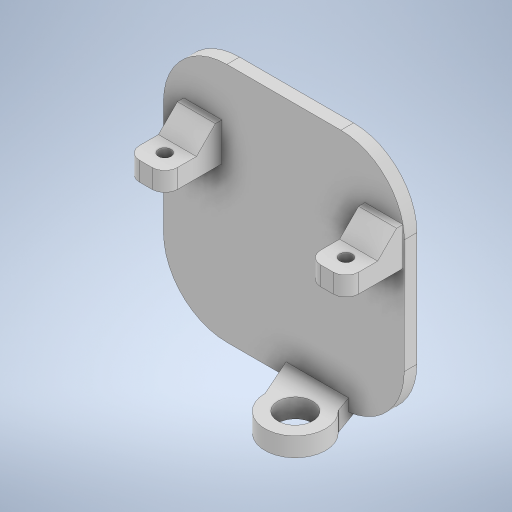
# Autodesk Inventor part: cabeza_nueva
Saved by Autodesk Inventor 2024 (Build 280153000, 153)
## iProperties
Created: 2025-05-13
Part Number: cabeza_nueva
Material: Genérico
Document SubType Name: Modeling
Designer: mario
Density: 1 g/cm^3
Appearance: Valor por defecto
Author: mario
Autodesk Inventor part; units mm, degrees
ref_plane "YZ Plane" through (0, 0, 0) normal (1, 0, 0) x (0, 1, 0)
ref_plane "XZ Plane" through (0, 0, 0) normal (0, 1, 0) x (-1, 0, 0)
ref_plane "XY Plane" through (0, 0, 0) normal (0, 0, 1) x (1, 0, 0)
sketch "Boceto3" plane through (-69.7362, 30.866, 0) normal (0, 0, -1) x (-1, 0, 0)
  line L0 (-8.7362, 5.134) -> (-26.7362, 5.134)
  line L1 (-36.7362, -4.866) -> (-36.7362, -22.866)
  line L2 (-26.7362, -32.866) -> (-8.7362, -32.866)
  line L3 (1.2638, -22.866) -> (1.2638, -4.866)
  line L4 (1.2638, -23.3279) -> (1.2638, -4.4042) construction
  line L5 (-8.2744, 5.134) -> (-27.1981, 5.134) construction
  line L6 (-36.7362, -4.4042) -> (-36.7362, -23.3295) projected
  circle A0 centre (-8.7362, -22.866) radius 10.0001 construction
  arc A1 (-8.7362, -32.866) -> (1.2638, -22.866) centre (-8.7362, -22.866) ccw
  arc A2 (1.2638, -4.866) -> (-8.7362, 5.134) centre (-8.7362, -4.866) ccw
  arc A3 (-26.7362, 5.134) -> (-36.7362, -4.866) centre (-26.7362, -4.866) ccw
  arc A4 (-36.7362, -22.866) -> (-26.7362, -32.866) centre (-26.7362, -22.866) ccw
  point P0 (-69.7362, -30.866)
  point P1 (1.2638, 5.134)
  point P2 (-36.7362, 5.134)
  dimension "d3" = 10
  dimension "d4" = 10
  constraints: 9 tangent, 8 end point, 8 point on circle, 7 point on line, 4 centre point, 2 equal radius, 2 parallel, 1 horizontal, 1 perpendicular
  measures "d3" radius of A1
  measures "d4" radius of A2
extrude "Extrusión2" add sketch "Boceto3" against normal blind 2
sketch "Boceto5" plane through (-61, -2, 0) normal (0, -1, 0) x (1, 0, 0)
  line L0 (18, 0) -> (28, 0) construction
  line L1 (18.5, 0) -> (20.0893, 4.4576)
  line L2 (20.0893, 4.4576) -> (12.0357, 8.0433)
  line L3 (12.0357, 8.0433) -> (8.4546, 0)
  line L4 (18, 0) -> (0, 0) construction
  line L5 (8.4546, 0) -> (18.5, 0)
  point P0 (61, 0)
  dimension "d7" = 9.5
  dimension "d8" = 66
  dimension "d9" = 8.8157
  dimension "d16" = 70.378
  dimension "d17" = 10.0454
  constraints: 8 end point, 2 point on line, 1 horizontal, 1 perpendicular
  measures "d7" distance of L1.start L0.end
  measures "d8" angle of L3 L4
  measures "d9" distance of L1.end L2.end
  measures "d16" angle of L1 L0
  measures "d17" distance of L3.end L1.start
extrude "Extrusión3" add sketch "Boceto5" along normal blind 1 and the other way blind 2
sketch "Boceto6" plane through (-61, -3, 0) normal (0, -1, 0) x (1, 0, 0)
  circle A0 centre (16.8, 8) radius 2.8 construction
  circle A1 centre (16.8003, 7.9997) radius 4.8004 projected
  point P0 (61, 0)
extrude "Extrusión4" add sketch "Boceto6" against normal blind 3
sketch "Boceto7" plane through (-61, -3, 0) normal (0, -1, 0) x (1, 0, 0)
  arc A0 (20.0563, 4.4723) -> (12, 7.9631) centre (16.8003, 7.9997) ccw projected
  point P0 (61, 0)
  constraints: 1 coincident
hole "Agujero1" at (-44.1997, -3, 7.9997) direction (0, 1, 0) diameter 5.5 end through all
sketch "Boceto8" plane through (-69.7362, 30.866, 2) normal (0, 0, 1) x (1, 0, 0)
  line L0 (36.5362, -8.866) -> (30.5362, -8.866)
  line L1 (30.5362, -8.866) -> (30.5362, -5.866)
  line L2 (30.5362, -5.866) -> (36.5362, -5.866)
  line L3 (36.5362, -5.866) -> (36.5362, -8.866)
  line L4 (36.7362, -22.866) -> (36.7362, -4.866) construction
  point P0 (69.7362, -30.866)
  dimension "d27" = 0.2
  dimension "d28" = 3
  dimension "d29" = 6
  dimension "d30" = 1
  constraints: 8 end point, 2 parallel, 1 horizontal, 1 perpendicular
  measures "d27" distance between parallel lines of L4 L3
  measures "d28" distance of L0.end L1.end
  measures "d29" distance of L0.start L0.end
  measures "d30" distance from line of L4.end L2
extrude "Extrusión5" add sketch "Boceto8" along normal blind 9
fillet "Empalme1" radius 2 2 edges at (-33.2, 23.5, 11) (-39.2, 23.5, 11)
sketch "Boceto9" plane through (-39.2, 22, 2) normal (0, -1, 0) x (1, 0, 0)
  line L0 (2, 9) -> (4, 9) construction
  line L1 (3, 9) -> (3, 0) construction
  line L2 (6, 0) -> (0, 0) construction
  point P0 (39.2, -2)
  point P1 (3, 6)
  dimension "d34" = 3
  constraints: 2 end point, 2 midpoint, 1 point on line
  measures "d34" distance from line of L0 point (3, 6)
hole "Agujero2" at (-36.2, 22, 8) direction (0, 1, 0) diameter 2 end through all
sketch "Boceto10" plane through (-33.2, 22, 2) normal (1, 0, 0) x (0, 0, -1)
  line L0 (0, 3) -> (-7, 3) construction
  line L1 (-4, 3) -> (-1, 6)
  line L2 (-1, 6) -> (0, 6)
  line L3 (0, 6) -> (0, 3)
  line L4 (-4, 3) -> (0, 3)
  point P0 (2, -22)
  dimension "d42" = 45
  dimension "d43" = 1
  dimension "d44" = 3
  constraints: 8 end point, 1 horizontal, 1 parallel, 1 perpendicular, 1 point on line
  measures "d42" angle of L1 L0
  measures "d43" distance of L1.end L2.end
  measures "d44" distance of L2.end L0.start
extrude "Extrusión6" add sketch "Boceto10" against normal blind 6
pattern_linear "Patrón rectangular1" count 2 spacing 28.6 along (-1, 0, 0) of "Extrusión6", "Extrusión5", "Agujero2", "Empalme1"
